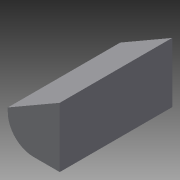
# Autodesk Inventor part: DMJ_Waist
Saved by Autodesk Inventor 2015 SP1 (Build 190203100, 203)
## iProperties
Created: 2016-02-03
Part Number: DMJ_Waist
Material: Generic
Document SubType Name: Modeling
Designer: guillemd
Density: 1 g/cm^3
Appearance: Default
Author: guillemd
Autodesk Inventor part; units mm, degrees
ref_plane "YZ Plane" through (0, 0, 0) normal (1, 0, 0) x (0, 1, 0)
ref_plane "XZ Plane" through (0, 0, 0) normal (0, 1, 0) x (-1, 0, 0)
ref_plane "XY Plane" through (0, 0, 0) normal (0, 0, 1) x (1, 0, 0)
sketch "Sketch1" plane through (0, 0, 0) normal (0, 0, 1) x (1, 0, 0)
  line L0 (0, 203.2) -> (0, 0)
  line L1 (0, 0) -> (-88.9, 0)
  line L2 (-175.9764, 101.6) -> (-175.9764, 87.0764)
  arc A0 (-175.9764, 87.0764) -> (-88.9, 0) centre (-88.9, 87.0764) ccw
  line L3 (-175.9764, 101.6) -> (0, 203.2)
  line L4 (0, -62.2809) -> (0, 247.4468) projected
  dimension "d1" = 203.2
  dimension "d2" = 60
  dimension "d3" = 203.2
  dimension "d4" = 88.9
  constraints: 8 end point, 2 perpendicular, 2 point on circle, 2 tangent, 1 centre point, 1 coincident, 1 horizontal, 1 point on line
  measures "d1" distance of L0.start L2.start
  measures "d2" angle of L0 L3
  measures "d3" distance of L0.start L0.end
  measures "d4" horizontal distance of point (0, 0) A0.centre
extrude "Extrusion1" add sketch "Sketch1" along normal mid plane 381
body "Solid1"
